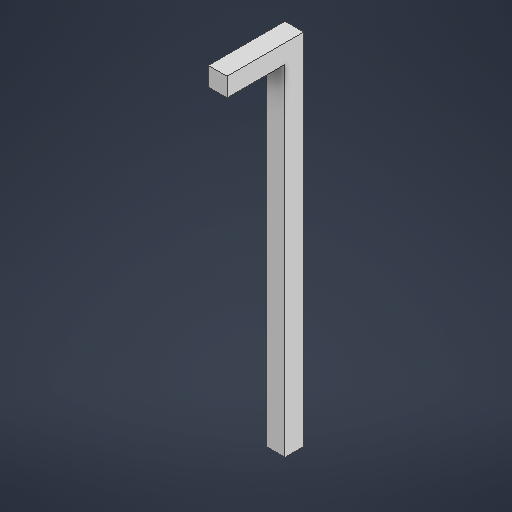
# Autodesk Inventor part: jst-vh-2p_wire
Saved by Autodesk Inventor 2025.2 (Build 292293000, 293)
## iProperties
Created: 2025-12-13
Part Number: jst-vh-2p_wire
Material: Generic
Document SubType Name: Modeling
Designer: sam
Density: 1 g/cm^3
Appearance: Default
Author: sam
Autodesk Inventor part; units mm, degrees
ref_plane "YZ Plane" through (0, 0, 0) normal (1, 0, 0) x (0, 1, 0)
ref_plane "XZ Plane" through (0, 0, 0) normal (0, 1, 0) x (-1, 0, 0)
ref_plane "XY Plane" through (0, 0, 0) normal (0, 0, 1) x (1, 0, 0)
sketch "Sketch4" plane through (0, 0, 0) normal (0, 1, 0) x (-1, 0, 0)
  line L0 (0.5, 0.5) -> (-0.5, 0.5)
  line L1 (-0.5, 0.5) -> (-0.5, -0.5)
  line L2 (-0.5, -0.5) -> (0.5, -0.5)
  line L3 (0.5, -0.5) -> (0.5, 0.5)
  line L4 (0.5, 0.5) -> (-0.5, -0.5) construction
  line L5 (-0.5, 0.5) -> (0.5, -0.5) construction
  point P0 (0, 0)
  dimension "d13" = 1
  dimension "d14" = 1
  constraints: 12 end point, 2 midpoint, 2 parallel, 1 horizontal, 1 perpendicular
  measures "d13" distance of L2.end L1.end
  measures "d14" distance of L1.end L0.end
extrude "Extrusion4" add sketch "Sketch4" along normal blind 19.2
sketch "Sketch5" plane through (-0.5, 0, 0.5) normal (0, 0, 1) x (1, 0, 0)
  line L0 (1, 19.2) -> (0, 19.2) projected
  line L1 (1, 0) -> (1, 19.2) projected
  line L2 (0, 19.2) -> (1, 19.2)
  line L3 (1, 19.2) -> (1, 18.2)
  line L4 (1, 18.2) -> (0, 18.2)
  line L5 (0, 18.2) -> (0, 19.2)
  point P0 (0.5, 0)
  dimension "d17" = 1
  constraints: 8 end point, 2 parallel, 1 horizontal, 1 perpendicular, 1 point on line
  measures "d17" distance of L2.end L3.end
extrude "Extrusion5" add sketch "Sketch5" along normal blind 3.1
body "Solid2"
